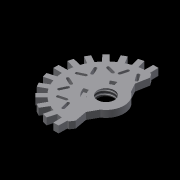
# Autodesk Inventor part: ShoulderCogLarge
Saved by Autodesk Inventor 2015 (Build 190159000, 159)
## iProperties
Created: 2014-09-25
Part Number: ShoulderCogLarge
Material: Generic
Document SubType Name: Modeling
Designer: Inventor
Mass: 0.605326 g
Surface Area: 10.3568 cm^2
Volume: 0.605326 cm^3
Density: 1 g/cm^3
Appearance: Default
Property Set Nam%: Inventor User Defined Properties
Author: Inventor
Autodesk Inventor part; units mm, degrees
ref_plane "YZ Plane" through (0, 0, 0) normal (1, 0, 0) x (0, 1, 0)
ref_plane "XZ Plane" through (0, 0, 0) normal (0, 1, 0) x (-1, 0, 0)
ref_plane "XY Plane" through (0, 0, 0) normal (0, 0, 1) x (1, 0, 0)
sketch "Body" plane through (0, 0, 0) normal (0, 0, 1) x (1, 0, 0)
  circle A0 centre (0, 0) radius 14.5 construction
  circle A1 centre (0, 0) radius 12
  line L0 (0, 0) -> (0, 14.5) construction
  line L1 (-0.75, 14.4806) -> (0.75, 14.4806)
  line L2 (-0.75, 14.4806) -> (-0.7938, 11.9737)
  line L3 (0.75, 14.4806) -> (0.7938, 11.9737)
  line L4 (-0.7938, 11.9737) -> (0.7938, 11.9737)
  point P0 (0, 14.4806)
  dimension "d0" = 29
  dimension "d1" = 2.5
  dimension "d2" = 1.5
  dimension "d3" = 91
  dimension "d4" = 91
  constraints: 10 end point, 4 point on circle, 2 centre point, 2 coincident, 1 horizontal, 1 midpoint, 1 point on line, 1 vertical
  measures "d0" diameter of A0
  measures "d1" radial gap between concentric circles of A0 A1
  measures "d2" distance of L1.start L1.end
  measures "d3" angle of L1 L2
  measures "d4" angle of L1 L3
extrude "BodyFeature" add sketch "Body" along normal blind 2 contours A1 L4 picked at (-0.413, -3.9477)
sketch "Tooth" plane through (0, 0, 0) normal (0, 0, -1) x (-1, 0, 0)
  line L0 (0.75, 14.4806) -> (0.7938, 11.9737) projected
  line L1 (0.75, 14.4806) -> (-0.75, 14.4806) projected
  line L2 (-0.75, 14.4806) -> (-0.7938, 11.9737) projected
  line L3 (0.7938, 11.9737) -> (-0.7938, 11.9737) projected
extrude "ToothFeature" add sketch "Tooth" against normal blind 2
pattern_circular "ToothArray" count 13 over 180 about axis through (0, 0, 0) along (0, 0, 1) of "ToothFeature"
sketch "Sketch3" plane through (0, 0, 0) normal (0, 0, -1) x (-1, 0, 0)
  point P0 (0, 0)
hole "BodyHole" at (0, 0, 0) direction (0, 0, 1) diameter 4.917 end through all thread size "M6x1" class "6H" standard "ISO Metric profile"
sketch "BodyCutDetail" plane through (0, 0, 2) normal (0, 0, 1) x (1, 0, 0)
  circle A0 centre (0, 0) radius 2.4585 construction
  line L0 (-6.6478, 7.2716) -> (-3.75, 6.4952) construction
  line L1 (-3.75, 6.4952) -> (-2.9735, 9.393) construction
  line L2 (-3.75, 6.4952) -> (0, 0) construction
  circle A1 centre (-2.9735, 9.393) radius 0.4
  circle A2 centre (-6.6478, 7.2716) radius 0.4
  circle A3 centre (-3.4912, 7.4611) radius 0.4
  circle A4 centre (-4.7159, 6.754) radius 0.4
  line L3 (-2.9735, 9.393) -> (-3.4912, 7.4611) construction
  line L4 (-4.7159, 6.754) -> (-6.6478, 7.2716) construction
  line L5 (-2.5872, 9.2894) -> (-3.1048, 7.3576)
  line L6 (-3.3599, 9.4965) -> (-3.8776, 7.5646)
  line L7 (-4.6124, 7.1404) -> (-6.5442, 7.658)
  line L8 (-4.8195, 6.3676) -> (-6.7513, 6.8853)
  line L9 (-3.75, 6.4952) -> (-7.2403, 12.5406) construction
  line L10 (-6.5908, 12.9156) -> (-7.8898, 12.1656) construction
  circle A5 centre (-8.3155, 5.2841) radius 0.4
  circle A6 centre (-9.7666, 1.2973) radius 0.4
  circle A7 centre (-7.4703, 3.4715) radius 0.4
  circle A8 centre (-7.954, 2.1425) radius 0.4
  line L11 (-7.953, 5.4531) -> (-7.1078, 3.6405)
  line L12 (-8.6781, 5.115) -> (-7.8328, 3.3024)
  line L13 (-8.123, 2.5051) -> (-9.9357, 1.6598)
  line L14 (-7.785, 1.78) -> (-9.5976, 0.9348)
  circle A9 centre (-9.7666, -1.2973) radius 0.4
  circle A10 centre (-8.3155, -5.2841) radius 0.4
  circle A11 centre (-7.954, -2.1425) radius 0.4
  circle A12 centre (-7.4703, -3.4715) radius 0.4
  line L15 (-9.5976, -0.9348) -> (-7.785, -1.78)
  line L16 (-9.9357, -1.6598) -> (-8.123, -2.5051)
  line L17 (-7.8328, -3.3024) -> (-8.6781, -5.115)
  line L18 (-7.1078, -3.6405) -> (-7.953, -5.4531)
  circle A13 centre (-6.6478, -7.2716) radius 0.4
  circle A14 centre (-2.9735, -9.393) radius 0.4
  circle A15 centre (-4.7159, -6.754) radius 0.4
  circle A16 centre (-3.4912, -7.4611) radius 0.4
  line L19 (-6.7513, -6.8853) -> (-4.8195, -6.3676)
  line L20 (-6.5442, -7.658) -> (-4.6124, -7.1404)
  line L21 (-3.8776, -7.5646) -> (-3.3599, -9.4965)
  line L22 (-3.1048, -7.3576) -> (-2.5872, -9.2894)
  circle A17 centre (-0.4184, -9.8435) radius 0.4
  circle A18 centre (3.7598, -9.1068) radius 0.4
  circle A19 centre (0.7288, -8.2052) radius 0.4
  circle A20 centre (2.1215, -7.9596) radius 0.4
  line L23 (-0.746, -9.6141) -> (0.4011, -7.9758)
  line L24 (-0.0907, -10.0729) -> (1.0564, -8.4346)
  line L25 (1.8921, -8.2873) -> (3.5304, -9.4344)
  line L26 (2.3509, -7.632) -> (3.9892, -8.7791)
  circle A21 centre (6.0068, -7.8095) radius 0.4
  circle A22 centre (8.7339, -4.5594) radius 0.4
  circle A23 centre (5.8325, -5.8171) radius 0.4
  circle A24 centre (6.7415, -4.7338) radius 0.4
  line L27 (5.6083, -7.8444) -> (5.434, -5.852)
  line L28 (6.4053, -7.7746) -> (6.231, -5.7822)
  line L29 (6.7764, -5.1322) -> (8.7688, -4.9579)
  line L30 (6.7067, -4.3353) -> (8.6991, -4.161)
  circle A25 centre (9.6213, -2.1213) radius 0.4
  circle A26 centre (9.6213, 2.1213) radius 0.4
  circle A27 centre (8.2071, -0.7071) radius 0.4
  circle A28 centre (8.2071, 0.7071) radius 0.4
  line L31 (9.3385, -2.4042) -> (7.9243, -0.9899)
  line L32 (9.9042, -1.8385) -> (8.4899, -0.4243)
  line L33 (8.4899, 0.4243) -> (9.9042, 1.8385)
  line L34 (7.9243, 0.9899) -> (9.3385, 2.4042)
  circle A29 centre (8.7339, 4.5594) radius 0.4
  circle A30 centre (6.0068, 7.8095) radius 0.4
  circle A31 centre (6.7415, 4.7338) radius 0.4
  circle A32 centre (5.8325, 5.8171) radius 0.4
  line L35 (8.6991, 4.161) -> (6.7067, 4.3353)
  line L36 (8.7688, 4.9579) -> (6.7764, 5.1322)
  line L37 (6.231, 5.7822) -> (6.4053, 7.7746)
  line L38 (5.434, 5.852) -> (5.6083, 7.8444)
  circle A33 centre (3.7598, 9.1068) radius 0.4
  circle A34 centre (-0.4184, 9.8435) radius 0.4
  circle A35 centre (2.1215, 7.9596) radius 0.4
  circle A36 centre (0.7288, 8.2052) radius 0.4
  line L39 (3.9892, 8.7791) -> (2.3509, 7.632)
  line L40 (3.5304, 9.4344) -> (1.8921, 8.2873)
  line L41 (1.0564, 8.4346) -> (-0.0907, 10.0729)
  line L42 (0.4011, 7.9758) -> (-0.746, 9.6141)
  dimension "d97" = 135
  dimension "d99" = 3
  dimension "d100" = 7.5
  dimension "d101" = 0.8
  dimension "d103" = 135
  dimension "d104" = 1
  dimension "d108" = 360
  constraints: 84 end point, 72 point on circle, 36 centre point, 8 tangent, 3 equal radius, 3 perpendicular, 2 coincident, 2 collinear, 1 midpoint, 181 other
  measures "d97" angle of L1 L2
  measures "d99" distance of L0.start L0.end
  measures "d100" distance of L0.end L2.end
  measures "d101" diameter of A1
  measures "d103" angle of L2 L0
  measures "d104" distance of L0.end L3.end
extrude "BodyCutDetailFeature" cut sketch "BodyCutDetail" against normal through all contours A1 | A1 L5 A3 L6 | A3 | A2 | A2 L7 A4 L8 | A4 | A5 | A5 L11 A7 L12 | A7 | A6 | A6 L13 A8 L14 | A8 | A9 | A9 L15 A11 L16 | A11 | A10 | A10 L17 A12 L18 | A12 | A13 | A13 L19 A15 L20 | A15 | A14 | A14 L21 A16 L22 | A16 | A17 | A17 L23 A19 L24 | A19 | A34 | A34 L41 A36 L42 | A36
sketch "CloseOneHole" plane through (0, 0, 0) normal (0, 0, -1) x (-1, 0, 0)
  circle A0 centre (-0.7288, -8.2052) radius 2.5
  arc A1 (-0.4011, -7.9758) -> (-1.0564, -8.4346) centre (-0.7288, -8.2052) ccw projected
  dimension "d153" = 5
  constraints: 1 centre point, 1 coincident
  measures "d153" diameter of A0
extrude "CloseOneHoleFeature" add sketch "CloseOneHole" against normal blind 2
sketch "BodyCutLimit" plane through (0, 0, 2) normal (0, 0, 1) x (1, 0, 0)
  circle A0 centre (0, 0) radius 2.4585 construction
  line L0 (0, 0) -> (2.1891, -11.7986) construction
  line L1 (0, 0) -> (2.1891, 11.7986) construction
  arc A1 (-5.2994, -10.7664) -> (0.7938, 11.9737) centre (0, 0) ccw construction
  circle A2 centre (0, 0) radius 5.25 construction
  arc A3 (2.1891, -11.7986) -> (2.1891, 11.7986) centre (0, 0) ccw
  arc A4 (0.9577, -5.1619) -> (0.9577, 5.1619) centre (0, 0) ccw
  line L2 (0.9577, -5.1619) -> (2.1891, -11.7986)
  line L3 (0.9577, 5.1619) -> (2.1891, 11.7986)
  point P0 (1.0564, -8.4346)
  point P1 (1.0564, 8.4346)
  dimension "d117" = 0.5
  dimension "d118" = 0.5
  dimension "d119" = 10.5
  constraints: 8 end point, 8 point on circle, 3 centre point, 2 concentric, 2 point on line, 1 coincident
  measures "d117" distance from line of L0 point (1.056, -8.435)
  measures "d118" distance from line of L1 point (1.056, 8.435)
  measures "d119" diameter of A2
extrude "BodyCutLimitFeature" cut sketch "BodyCutLimit" against normal through all
chamfer "BodyChamfer1Feature" distance 2 angle 45 1 edges at (0.9577, 5.1619, 1)
chamfer "BodyChamfer2Feature" distance 2 angle 45 1 edges at (0.9577, -5.1619, 1)
chamfer "BodyChamfer3Feature" distance 1 angle 45 1 edges at (2.1891, -11.7986, 1)
chamfer "BodyChamfer4Feature" distance 1 angle 45 1 edges at (2.1891, 11.7986, 1)
sketch "BodyDetail" plane through (0, 0, 2) normal (0, 0, 1) x (1, 0, 0)
  circle A0 centre (0, 0) radius 4 construction
  circle A1 centre (0, 0) radius 5.25 construction
  circle A2 centre (0, 0) radius 2.4585 construction
  line L0 (-2.966, -4.3319) -> (0, 0) construction
  line L1 (0, 0) -> (-5.0338, -1.4912) construction
  line L2 (2.8187, -4.4292) -> (1.3226, -7.1283) construction
  arc A3 (-5.0338, -1.4912) -> (-2.966, -4.3319) centre (0, 0) ccw
  arc A4 (-3.8352, -1.1362) -> (-2.2598, -3.3005) centre (0, 0) ccw
  line L3 (-5.0338, -1.4912) -> (-3.8352, -1.1362)
  line L4 (-2.966, -4.3319) -> (-2.2598, -3.3005)
  line L5 (0, 0) -> (-3.1229, 4.2202) construction
  line L6 (0, 0) -> (-1.666, 4.9787) construction
  arc A5 (-1.666, 4.9787) -> (-3.1229, 4.2202) centre (0, 0) ccw
  arc A6 (-1.2693, 3.7933) -> (-2.3794, 3.2154) centre (0, 0) ccw
  line L7 (-3.1229, 4.2202) -> (-2.3794, 3.2154)
  line L8 (-1.2693, 3.7933) -> (-1.666, 4.9787)
  dimension "d140" = 8
  dimension "d142" = 5.4
  dimension "d143" = 39.1
  dimension "d144" = 18
  dimension "d145" = 70
  constraints: 17 point on circle, 16 end point, 6 centre point, 5 concentric, 4 point on line, 2 collinear, 1 coincident
  measures "d140" diameter of A0
  measures "d142" angle of L0 L2
  measures "d143" angle of L1 L0
  measures "d144" angle of L6 L5
  measures "d145" angle of L5 L1
extrude "BodyDetailFeature" cut sketch "BodyDetail" against normal blind 1
equation "\"d4\" = d3"
equation "\"d103\" = d97"
